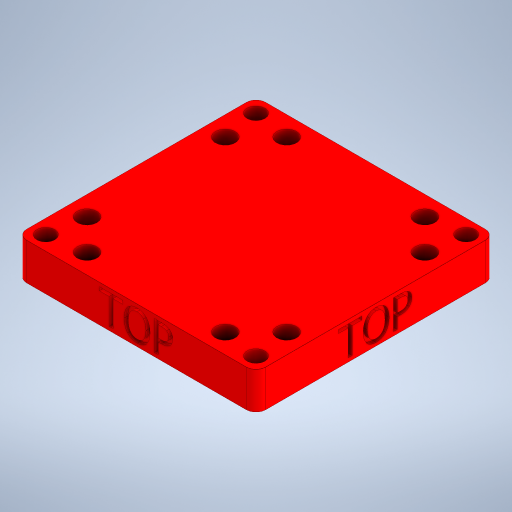
# Autodesk Inventor part: Cube 1x1 Top V5 Closed
Saved by Autodesk Inventor 2023.1 (Build 271208000, 208)
## iProperties
Created: 2022-07-25
Part Number: Cube 1x1 Top V5 Closed
Material: Generic
Document SubType Name: Modeling
Designer: xSibe
Density: 1 g/cm^3
Appearance: Plastic Red
Author: xSibe
Autodesk Inventor part; units mm, degrees
ref_plane "YZ Plane" through (0, 0, 0) normal (1, 0, 0) x (0, 1, 0)
ref_plane "XZ Plane" through (0, 0, 0) normal (0, 1, 0) x (-1, 0, 0)
ref_plane "XY Plane" through (0, 0, 0) normal (0, 0, 1) x (1, 0, 0)
sketch "Sketch1" plane through (0, 0, 0) normal (0, 1, 0) x (-1, 0, 0)
  line L0 (24.9, 24.9) -> (-24.9, 24.9)
  line L1 (-24.9, 24.9) -> (-24.9, -24.9)
  line L2 (-24.9, -24.9) -> (24.9, -24.9)
  line L3 (24.9, -24.9) -> (24.9, 24.9)
  line L4 (24.9, 24.9) -> (-24.9, -24.9) construction
  line L5 (-24.9, 24.9) -> (24.9, -24.9) construction
  line L6 (17.05, 17.05) -> (-17.05, 17.05)
  line L7 (-17.05, 17.05) -> (-17.05, -17.05)
  line L8 (-17.05, -17.05) -> (17.05, -17.05)
  line L9 (17.05, -17.05) -> (17.05, 17.05)
  line L10 (24.9, -24.9) -> (21.9, -24.9)
  line L11 (21.9, -24.9) -> (21.9, -21.9)
  line L12 (21.9, -21.9) -> (24.9, -21.9)
  line L13 (24.9, -21.9) -> (24.9, -24.9)
  circle A0 centre (21.9, -21.9) radius 1.875
  circle A1 centre (21.9, -21.9) radius 2.1063
  circle A2 centre (21.9, -21.9) radius 2.7813
  line L14 (24.9, -24.9) -> (14.4, -24.9)
  line L15 (14.4, -24.9) -> (14.4, -14.4)
  line L16 (14.4, -14.4) -> (24.9, -14.4)
  line L17 (24.9, -14.4) -> (24.9, -24.9)
  line L18 (24.9, -14.4) -> (20.8, -14.4)
  circle A3 centre (20.8, -14.4) radius 2.0734
  circle A4 centre (14.4, -20.8) radius 2.0734
  line L19 (24.9, -24.9) -> (17.05, -24.9)
  line L20 (17.05, -24.9) -> (17.05, -22.55)
  line L21 (22.55, -17.05) -> (24.9, -17.05)
  line L22 (24.9, -17.05) -> (24.9, -24.9)
  line L23 (22.55, -17.05) -> (17.05, -22.55)
  circle A5 centre (21.9, 21.9) radius 2.7813
  circle A6 centre (21.9, 21.9) radius 2.1063
  circle A7 centre (21.9, 21.9) radius 1.875
  circle A8 centre (14.4, 20.8) radius 2.0734
  circle A9 centre (20.8, 14.4) radius 2.0734
  line L24 (17.05, 22.55) -> (22.55, 17.05)
  line L25 (24.9, 17.05) -> (22.55, 17.05)
  line L26 (17.05, 22.55) -> (17.05, 24.9)
  circle A10 centre (-21.9, 21.9) radius 2.7813
  circle A11 centre (-21.9, 21.9) radius 2.1063
  circle A12 centre (-21.9, 21.9) radius 1.875
  circle A13 centre (-20.8, 14.4) radius 2.0734
  circle A14 centre (-14.4, 20.8) radius 2.0734
  line L27 (-22.55, 17.05) -> (-17.05, 22.55)
  line L28 (-17.05, 24.9) -> (-17.05, 22.55)
  line L29 (-22.55, 17.05) -> (-24.9, 17.05)
  circle A15 centre (-21.9, -21.9) radius 2.7813
  circle A16 centre (-21.9, -21.9) radius 2.1063
  circle A17 centre (-21.9, -21.9) radius 1.875
  circle A18 centre (-14.4, -20.8) radius 2.0734
  circle A19 centre (-20.8, -14.4) radius 2.0734
  line L30 (-17.05, -22.55) -> (-22.55, -17.05)
  line L31 (-24.9, -17.05) -> (-22.55, -17.05)
  line L32 (-17.05, -22.55) -> (-17.05, -24.9)
  line L33 (17.05, -22.55) -> (-17.05, -22.55)
  line L34 (-22.55, -17.05) -> (-22.55, 17.05)
  line L35 (-17.05, 22.55) -> (17.05, 22.55)
  line L36 (22.55, 17.05) -> (22.55, -17.05)
  point P0 (0, 0)
  point P1 (-15.5119, -22.55)
  point P2 (14.4, -22.8734)
  point P3 (13.2881, -22.55)
  point P4 (-13.2881, -22.55)
  point P5 (-22.55, -15.5119)
  point P6 (-22.55, -13.2881)
  point P7 (-22.55, 13.2881)
  point P8 (-22.55, 15.5119)
  point P9 (-15.5119, 22.55)
  point P10 (-13.2881, 22.55)
  point P11 (13.2881, 22.55)
  point P12 (15.5119, 22.55)
  point P13 (22.55, -15.5119)
  point P14 (22.55, 15.5119)
  point P15 (22.55, 13.2881)
  point P16 (22.55, -13.2881)
  point P17 (15.5119, -22.55)
  dimension "d0" = 49.8
  dimension "d1" = 49.8
  dimension "d2" = 7.85
  dimension "d3" = 3
  dimension "d4" = 3
  dimension "d5" = 3.75
  dimension "d6" = 4.2125
  dimension "d7" = 0.675
  dimension "d8" = 10.5
  dimension "d9" = 10.5
  dimension "d10" = 4.1
  dimension "d11" = 4.1467
  dimension "d12" = 7.85
  dimension "d13" = 7.85
  dimension "d14" = 5.5
  dimension "d15" = 5.5
  dimension "d18" = 360
  constraints: 74 end point, 20 centre point, 10 parallel, 7 perpendicular, 6 coincident, 4 horizontal, 3 point on line, 2 midpoint, 1 symmetric about line, 69 other
  measures "d0" distance of L2.end L1.end
  measures "d1" distance of L1.end L0.end
  measures "d2" distance between parallel lines of L3 L9
  measures "d3" distance of L11.end L12.end
  measures "d4" distance of L10.end L11.end
  measures "d5" diameter of A0
  measures "d6" diameter of A1
  measures "d7" radial gap between concentric circles of A1 A2
  measures "d8" distance of L15.end L16.end
  measures "d9" distance of L14.end L15.end
  measures "d10" distance of L16.end L18.end
  measures "d11" diameter of A3
  measures "d12" distance of point (17.05, -17.05) L21.end
  measures "d13" distance of L19.end point (17.05, -17.05)
  measures "d14" distance of L21.start point (17.05, -17.05)
  measures "d15" distance of L20.end point (17.05, -17.05)
extrude "Extrusion1" add sketch "Sketch1" along normal blind 7.7 contours L3 L25 L24 L26 L0 | L26 L35 A8 A14 L28 L0 | L3 L16 A3 L36 A9 L25 | L28 L27 L29 L1 L0 | L3 L21 L36 A3 L16 | L3 L12 A2 L11 L2 L20 L23 L21 | L29 L34 A13 A19 L31 L1 | L3 L2 L11 A2 L12 | L31 L30 L32 L2 L1 | A2 L11 A1 L12 | L12 A1 L11 A2 | L20 L2 L15 A4 L33 | A1 L11 A0 L12 | L12 A0 L11 A1 | L32 L33 A18 A4 L15 L2 | A0 L11 L12 | L12 L11 A0 | A5 | A6 | A7 | A10 | A11 | A12 | A15 | A16 | A17
extrude "Extrusion2" add sketch "Sketch1" against normal up to surface (7.7 mm away) from surface at 7.7 contours L26 L35 A8 A14 L28 L0 | L3 L16 A3 L36 A9 L25 | L24 L36 A9 A3 L16 L9 L6 L7 L8 L15 A4 L33 A18 L30 L34 A19 A13 L27 L35 A14 A8 | L3 L21 L36 A3 L16 | L29 L34 A13 A19 L31 L1 | L23 L33 A4 L15 L8 L9 L16 A3 L36 | L20 L2 L15 A4 L33 | L32 L33 A18 A4 L15 L2
chamfer "Chamfer1" [suppressed]
fillet "Fillet1" radius 2 4 edges at (24.9, 3.85, 24.9) (24.9, 3.85, -24.9) (-24.9, 3.85, -24.9) (-24.9, 3.85, 24.9)
chamfer "Chamfer2" distance 0.025 angle 45 16 edges at (19.975, 7.7, 24.9) (0, 7.7, 24.9) (-19.975, 7.7, 24.9) (24.3142, 7.7, 24.3142) (24.9, 7.7, -19.975) (24.9, 7.7, 0) (24.9, 7.7, 19.975) (24.3142, 7.7, -24.3142) (19.975, 7.7, -24.9) (0, 7.7, -24.9) (-19.975, 7.7, -24.9) (-24.3142, 7.7, -24.3142) (-24.9, 7.7, -19.975) (-24.9, 7.7, 19.975) (-24.9, 7.7, 0) (-24.3142, 7.7, 24.3142)
extrude "Extrusion3" cut sketch "Sketch1" along normal blind 3 contours A1 L11 A0 L12 | L12 A0 L11 A1 | A0 L11 L12 | L12 L11 A0 | A6 | A7 | A11 | A12 | A16 | A17
extrude "Extrusion4" cut sketch "Sketch1" along normal up to surface (4.7 mm away) from surface at 3 contours A0 L11 L12 | L12 L11 A0 | A7 | A12 | A17
sketch "Sketch2" plane through (0, 7.7, 24.9) normal (0, 0, 1) x (1, 0, 0)
  line L0 (-8.2534, -7.5059) -> (8.2534, -7.5059) construction
  line L1 (8.2534, -7.5059) -> (8.2534, -0.2191) construction
  line L2 (8.2534, -0.2191) -> (-8.2534, -0.2191) construction
  line L3 (-8.2534, -0.2191) -> (-8.2534, -7.5059) construction
  line L4 (-22.9, -3.8625) -> (22.9, -3.8625)
  line L5 (-8.2534, -3.8625) -> (8.2534, -3.8625)
  line L6 (-22.9, -0.025) -> (22.9, -0.025) projected
  line L7 (-22.9, -7.7) -> (-22.9, -0.025) projected
  line L8 (-22.9, -7.7) -> (22.9, -7.7) projected
  line L9 (22.9, -0.025) -> (22.9, -7.7) projected
  line L10 (-5.6897, -6.9125) -> (-5.6897, -1.5342)
  line L11 (-5.6897, -1.5342) -> (-7.7362, -1.5342)
  line L12 (-7.7362, -1.5342) -> (-7.7362, -0.8125)
  line L13 (-7.7362, -0.8125) -> (-2.8325, -0.8125)
  line L14 (-2.8325, -0.8125) -> (-2.8325, -1.5342)
  line L15 (-2.8325, -1.5342) -> (-4.879, -1.5342)
  line L16 (-4.879, -1.5342) -> (-4.879, -6.9125)
  line L17 (-4.879, -6.9125) -> (-5.6897, -6.9125)
  spline S0 degree 2 poles (2.1009, -1.5095) (2.4469, -1.9148) (2.8325, -3.1012) (2.8325, -3.8625) knots 0 0 0 1 2 2 2
  spline S1 degree 2 poles (2.8325, -3.8625) (2.8325, -4.604) (2.4568, -5.8052) (2.1009, -6.2106) knots 0 0 0 1 2 2 2
  spline S2 degree 2 poles (2.1009, -6.2106) (1.7252, -6.6357) (0.7316, -7.041) (0.1335, -7.041) knots 0 0 0 1 2 2 2
  spline S3 degree 2 poles (0.1335, -7.041) (-0.4844, -7.041) (-1.4731, -6.6208) (-1.834, -6.2106) knots 0 0 0 1 2 2 2
  spline S4 degree 2 poles (-1.834, -6.2106) (-2.1849, -5.8052) (-2.5606, -4.6139) (-2.5606, -3.8625) knots 0 0 0 1 2 2 2
  spline S5 degree 2 poles (-2.5606, -3.8625) (-2.5606, -3.0963) (-2.18, -1.9297) (-1.829, -1.5095) knots 0 0 0 1 2 2 2
  spline S6 degree 2 poles (-1.829, -1.5095) (-1.4731, -1.1042) (-0.4795, -0.684) (0.1335, -0.684) knots 0 0 0 1 2 2 2
  spline S7 degree 2 poles (0.1335, -0.684) (0.7563, -0.684) (1.7549, -1.119) (2.1009, -1.5095) knots 0 0 0 1 2 2 2
  spline S8 degree 2 poles (1.9872, -3.8625) (1.9872, -3.2594) (1.7252, -2.3251) (1.4879, -2.0187) knots 0 0 0 1 2 2 2
  spline S9 degree 2 poles (1.4879, -2.0187) (1.2457, -1.7023) (0.5635, -1.3859) (0.1384, -1.3859) knots 0 0 0 1 2 2 2
  spline S10 degree 2 poles (0.1384, -1.3859) (-0.3015, -1.3859) (-0.9639, -1.6924) (-1.216, -2.0187) knots 0 0 0 1 2 2 2
  spline S11 degree 2 poles (-1.216, -2.0187) (-1.4583, -2.3301) (-1.7153, -3.2693) (-1.7153, -3.8625) knots 0 0 0 1 2 2 2
  spline S12 degree 2 poles (-1.7153, -3.8625) (-1.7153, -5.0637) (-0.7069, -6.3391) (0.1384, -6.3391) knots 0 0 0 1 2 2 2
  spline S13 degree 2 poles (0.1384, -6.3391) (0.9837, -6.3391) (1.9872, -5.0637) (1.9872, -3.8625) knots 0 0 0 1 2 2 2
  spline S14 degree 2 poles (7.578, -2.6514) (7.578, -3.0469) (7.2963, -3.7587) (7.0442, -4.0059) knots 0 0 0 1 2 2 2
  spline S15 degree 2 poles (7.0442, -4.0059) (6.7278, -4.3173) (5.8726, -4.6386) (5.2201, -4.6386) knots 0 0 0 1 2 2 2
  line L18 (5.2201, -4.6386) -> (4.533, -4.6386)
  line L19 (4.533, -4.6386) -> (4.533, -6.9125)
  line L20 (4.533, -6.9125) -> (3.7223, -6.9125)
  line L21 (3.7223, -6.9125) -> (3.7223, -0.8125)
  line L22 (3.7223, -0.8125) -> (5.2547, -0.8125)
  spline S16 degree 2 poles (5.2547, -0.8125) (5.7985, -0.8125) (6.5597, -0.9905) (6.8514, -1.1931) knots 0 0 0 1 2 2 2
  spline S17 degree 2 poles (6.8514, -1.1931) (7.1925, -1.4255) (7.578, -2.1422) (7.578, -2.6514) knots 0 0 0 1 2 2 2
  spline S18 degree 2 poles (6.7327, -2.6761) (6.7327, -2.3597) (6.5152, -1.8951) (6.2928, -1.7468) knots 0 0 0 1 2 2 2
  spline S19 degree 2 poles (6.2928, -1.7468) (6.1, -1.6183) (5.5859, -1.5144) (5.2053, -1.5144) knots 0 0 0 1 2 2 2
  line L23 (5.2053, -1.5144) -> (4.533, -1.5144)
  line L24 (4.533, -1.5144) -> (4.533, -3.9465)
  line L25 (4.533, -3.9465) -> (5.0866, -3.9465)
  spline S20 degree 2 poles (5.0866, -3.9465) (5.581, -3.9465) (6.189, -3.7884) (6.3867, -3.5807) knots 0 0 0 1 2 2 2
  spline S21 degree 2 poles (6.3867, -3.5807) (6.5696, -3.3978) (6.7327, -2.9678) (6.7327, -2.6761) knots 0 0 0 1 2 2 2
  point P0 (0, -7.7)
  point P1 (0, -3.8625)
  constraints: 6 midpoint, 4 end point, 1 horizontal, 2 other
extrude "Extrusion5" cut sketch "Sketch2" against normal blind 0.75 contours L10 L11 L12 L13 L14 L15 L16 L4 | L4 L16 L17 L10 | S5 S6 S7 S0 L4 S8 S9 S10 S11 | L4 S12 S13 S1 S2 S3 S4 | S14 S15 L18 L19 L20 L21 L4 L24 L25 S20 | L4 S20 S21 S18 S19 L23 L24 L21 L22 S16 S17 S14
pattern_circular "Circular Pattern1" count 4 over 360 about axis through (0, -10, 0) along (0, 1, 0) of "Extrusion5"
sketch "Sketch3" plane through (0, 7.7, 0) normal (0, 1, 0) x (1, 0, 0)
  circle A0 centre (21.9, 21.9) radius 1.875 projected
  circle A1 centre (-21.9, -21.9) radius 1.875 projected
  circle A2 centre (-21.9, 21.9) radius 1.875 projected
  circle A3 centre (21.9, -21.9) radius 1.875 projected
  circle A4 centre (-14.4, -20.8) radius 2.0734 projected
  circle A5 centre (14.4, 20.8) radius 2.0734 projected
  circle A6 centre (-14.4, 20.8) radius 2.0734 projected
  circle A7 centre (-20.8, 14.4) radius 2.0734 projected
  line L0 (17.05, -17.05) -> (17.05, 17.05) projected
  line L1 (-17.05, -17.05) -> (17.05, -17.05) projected
  line L2 (-17.05, 17.05) -> (-17.05, -17.05) projected
  line L3 (17.05, 17.05) -> (-17.05, 17.05) projected
  circle A8 centre (-20.8, -14.4) radius 2.0734 projected
  circle A9 centre (14.4, -20.8) radius 2.0734 projected
  circle A10 centre (20.8, 14.4) radius 2.0734 projected
  circle A11 centre (20.8, -14.4) radius 2.0734 projected
  line L4 (22.9, -24.875) -> (-22.9, -24.875) projected
  arc A12 (22.9, -24.875) -> (24.875, -22.9) centre (22.9, -22.9) ccw projected
  line L5 (24.875, 22.9) -> (24.875, -22.9) projected
  arc A13 (24.875, 22.9) -> (22.9, 24.875) centre (22.9, 22.9) ccw projected
  line L6 (-22.9, 24.875) -> (22.9, 24.875) projected
  arc A14 (-22.9, 24.875) -> (-24.875, 22.9) centre (-22.9, 22.9) ccw projected
  line L7 (-24.875, -22.9) -> (-24.875, 22.9) projected
  arc A15 (-24.875, -22.9) -> (-22.9, -24.875) centre (-22.9, -22.9) ccw projected
  point P0 (0, 0)
extrude "Extrusion6" add sketch "Sketch3" against normal blind 2.2 contours L1 L2 L3 L0
equation "\"d15\" = d14"
body "Solid1"
